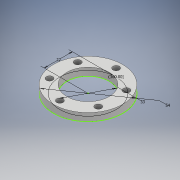
# Autodesk Inventor part: SpacerSprocketHubPlate
Saved by Autodesk Inventor 2019.3 (Build 233278000, 278)
## iProperties
Created: 2017-05-06
Part Number: SpacerSprocketHubPlate
Material: Generic
Document SubType Name: Modeling
Designer: eroldan
Density: 1 g/cm^3
Appearance: Default
Author: eroldan
Autodesk Inventor part; units mm, degrees
ref_plane "YZ Plane" through (0, 0, 0) normal (1, 0, 0) x (0, 1, 0)
ref_plane "XZ Plane" through (0, 0, 0) normal (0, 1, 0) x (-1, 0, 0)
ref_plane "XY Plane" through (0, 0, 0) normal (0, 0, 1) x (1, 0, 0)
sketch "Sketch1" plane through (0, 0, 0) normal (0, 0, 1) x (1, 0, 0)
  circle A0 centre (0, 0) radius 16.5
  circle A1 centre (0, 0) radius 27
  point P0 (0, 22)
  point P1 (-19.0526, 11)
  point P2 (-19.0526, -11)
  point P3 (0, -22)
  point P4 (19.0526, -11)
  point P5 (19.0526, 11)
  dimension "d9" = 33
  dimension "d20" = 22
  dimension "d23" = 360
  dimension "d58" = 54
  constraints: 2 centre point, 1 coincident, 7 other
  measures "d9" diameter of A0
  measures "d20" distance of point (0, 22) point (0, 0)
  measures "d58" diameter of A1
extrude "Extrusion2" add sketch "Sketch1" along normal blind 6
hole "Hole3" at (0, 22, 0) at (-19.0526, 11, 0) at (-19.0526, -11, 0) at (0, -22, 0) at (19.0526, 11, 0) at (19.0526, -11, 0) direction (0, 0, 1) diameter 5 end through all
